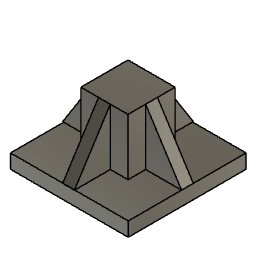
3D Plancha 8 (Autodesk Fusion 360 design; units mm, degrees)
Autodesk Fusion 360 part; units mm, degrees
sketch "Boceto1" plane through (0, 0, 0) normal (0, 0, 1) x (1, 0, 0)
  line L0 (0.4387, 129.7923) -> (100.4387, 129.7923)
  line L1 (100.4387, 129.7923) -> (100.4387, 29.7923)
  line L2 (100.4387, 29.7923) -> (0.4387, 29.7923)
  line L3 (0.4387, 29.7923) -> (0.4387, 129.7923)
  line L4 (30, 100) -> (70, 100)
  line L5 (70, 100) -> (70, 60)
  line L6 (70, 60) -> (30, 60)
  line L7 (30, 60) -> (30, 100)
  line L8 (50.4387, 29.7923) -> (50.4387, 27.3857)
  point P0 (50.4387, 79.7923)
  point P1 (50.4387, 79.7923)
  point P2 (50.4387, 79.7923)
  point P3 (50.4387, 79.7923)
  point P4 (50.4387, 79.7923)
  point P5 (50.4387, 74.7923)
  constraint horizontal L0
  constraint vertical L1
  constraint horizontal L2
  constraint vertical L3
  constraint horizontal L4
  constraint vertical L5
  constraint horizontal L6
  constraint vertical L7
  constraint coincident L2 L8.start
extrude "Extruir1" add sketch "Boceto1" along normal blind 12 makes body 1
extrude "Extruir2" add sketch "Boceto1" along normal blind 60 contours L4 L5 L6 L7 bodies 1
sketch "Boceto2" plane through (0, 0, 0) normal (0, 1, 0) x (1, 0, 0)
  line L0 (70, -60) -> (100.44, -12)
  line L1 (100.44, -12) -> (70, -12)
  line L2 (70, -12) -> (70, -60)
  constraint horizontal L1
  constraint perpendicular L1 L2
extrude "Extruir3" add sketch "Boceto2" along normal blind 10 separate body makes body 2
copy_body "CopiarPegarCuerpos1" bodies 2 makes body 3
move_body "Desplazar1" bodies 3 to x (1, 0, 0) y (0, 1, 0) z (0, 0, 1) at (-55.0952, -40.3111, 14.7841)
copy_body "CopiarPegarCuerpos2" bodies 2 makes body 4
move_body "Desplazar2" bodies 4 to x (1, 0, 0) y (0, 1, 0) z (0, 0, 1) at (82.6793, 90.7867, 8.1074)
copy_body "CopiarPegarCuerpos3" bodies 2 makes body 5
move_body "Desplazar3" bodies 5 to x (1, 0, 0) y (0, 1, 0) z (0, 0, 1) at (7.8026, 85.5386, 77.736)
move_body "Alinear1" bodies 5 to x (1, 0, 0) y (0, 1, 0) z (0, 0, 1) at (-7.8026, -10.5386, -77.736)
move_body "Alinear2" bodies 4 to x (0, 1, 0) y (-1, 0, 0) z (0, 0, 1) at (145.7867, -52.6793, -8.1074)
move_body "Alinear3" bodies 2 to x (-1, 0, 0) y (0, -1, 0) z (0, 0, 1) at (100, 85, 0)
move_body "Alinear4" bodies 3 to x (0, -1, 0) y (1, 0, 0) z (0, 0, 1) at (85.3111, 74.9048, -14.7841)
